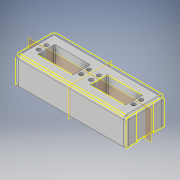
# Autodesk Inventor part: Socle servo
Saved by Autodesk Inventor 2018 (Build 220112000, 112)
## iProperties
Created: 2017-10-12
Part Number: Socle servo
Material: Generic
Document SubType Name: Modeling
Designer: liamg
Density: 1 g/cm^3
Appearance: Default
Author: liamg
Autodesk Inventor part; units mm, degrees
ref_plane "XZ Plane" through (0, 0, 0) normal (0, 1, 0) x (-1, 0, 0)
sketch "Sketch1" plane through (0, 0, 0) normal (0, 1, 0) x (-1, 0, 0)
  line L0 (-10.577, 9.85) -> (-48.827, 9.85) construction
  arc A0 (-9.577, 8.85) -> (-10.577, 9.85) centre (-10.577, 8.85) ccw construction
  line L1 (-9.577, -8.85) -> (-9.577, 8.85) construction
  arc A1 (-10.577, -9.85) -> (-9.577, -8.85) centre (-10.577, -8.85) ccw construction
  line L2 (-48.827, -9.85) -> (-10.577, -9.85) construction
  arc A2 (-49.827, -8.85) -> (-48.827, -9.85) centre (-48.827, -8.85) ccw construction
  line L3 (-49.827, 8.85) -> (-49.827, -8.85) construction
  arc A3 (-48.827, 9.85) -> (-49.827, 8.85) centre (-48.827, 8.85) ccw construction
  circle A4 centre (-19.427, 0) radius 6.44 construction
  circle A5 centre (-19.427, 0) radius 5.44 construction
  line L4 (-9.577, 9.475) -> (-3.217, 9.475) construction
  arc A6 (-2.217, 8.475) -> (-3.217, 9.475) centre (-3.217, 8.475) ccw construction
  line L5 (-2.217, -8.475) -> (-2.217, 8.475) construction
  arc A7 (-3.217, -9.475) -> (-2.217, -8.475) centre (-3.217, -8.475) ccw construction
  line L6 (-9.577, -9.475) -> (-3.217, -9.475) construction
  circle A8 centre (-5.6393, -4.36) radius 2.3 construction
  circle A9 centre (-5.6393, 4.36) radius 2.18 construction
  line L7 (-49.6076, 9.475) -> (-56.187, 9.475) construction
  arc A10 (-56.187, 9.475) -> (-57.187, 8.475) centre (-56.187, 8.475) ccw construction
  line L8 (-57.187, -8.475) -> (-57.187, 8.475) construction
  circle A11 centre (-53.7647, 4.36) radius 2.18 construction
  circle A12 centre (-53.7647, -4.36) radius 2.3 construction
  line L9 (-56.187, -9.475) -> (-49.6076, -9.475) construction
  arc A13 (-57.187, -8.475) -> (-56.187, -9.475) centre (-56.187, -8.475) ccw construction
  line L10 (48.9003, 9.85) -> (10.6503, 9.85) construction
  arc A14 (49.9003, 8.85) -> (48.9003, 9.85) centre (48.9003, 8.85) ccw construction
  line L11 (49.9003, -8.85) -> (49.9003, 8.85) construction
  arc A15 (48.9003, -9.85) -> (49.9003, -8.85) centre (48.9003, -8.85) ccw construction
  line L12 (10.6503, -9.85) -> (48.9003, -9.85) construction
  arc A16 (9.6503, -8.85) -> (10.6503, -9.85) centre (10.6503, -8.85) ccw construction
  line L13 (9.6503, 8.85) -> (9.6503, -8.85) construction
  arc A17 (10.6503, 9.85) -> (9.6503, 8.85) centre (10.6503, 8.85) ccw construction
  circle A18 centre (40.0503, 0) radius 6.44 construction
  circle A19 centre (40.0503, 0) radius 5.44 construction
  line L14 (49.9003, 9.475) -> (56.2603, 9.475) construction
  arc A20 (57.2603, 8.475) -> (56.2603, 9.475) centre (56.2603, 8.475) ccw construction
  line L15 (57.2603, -8.475) -> (57.2603, 8.475) construction
  arc A21 (56.2603, -9.475) -> (57.2603, -8.475) centre (56.2603, -8.475) ccw construction
  line L16 (49.9003, -9.475) -> (56.2603, -9.475) construction
  circle A22 centre (53.838, -4.36) radius 2.3 construction
  circle A23 centre (53.838, 4.36) radius 2.18 construction
  line L17 (9.8697, 9.475) -> (3.2903, 9.475) construction
  arc A24 (3.2903, 9.475) -> (2.2903, 8.475) centre (3.2903, 8.475) ccw construction
  line L18 (2.2903, -8.475) -> (2.2903, 8.475) construction
  circle A25 centre (5.7126, 4.36) radius 2.18 construction
  circle A26 centre (5.7126, -4.36) radius 2.3 construction
  line L19 (3.2903, -9.475) -> (9.8697, -9.475) construction
  arc A27 (2.2903, -8.475) -> (3.2903, -9.475) centre (3.2903, -8.475) ccw construction
  line L20 (-62.7873, 21.97) -> (62.7873, 21.97)
  line L21 (62.7873, 21.97) -> (62.7873, -21.97)
  line L22 (62.7873, -21.97) -> (-62.7873, -21.97)
  line L23 (-62.7873, -21.97) -> (-62.7873, 21.97)
  line L24 (-62.7873, 21.97) -> (62.7873, -21.97) construction
  line L25 (62.7873, 21.97) -> (-62.7873, -21.97) construction
  point P0 (0, 0)
  constraints: 52 end point, 32 point on circle, 28 centre point, 2 midpoint, 2 parallel, 1 horizontal, 1 perpendicular
extrude "Socle" add sketch "Sketch1" along normal blind 30
sketch "Sketch2" plane through (0, 30, 0) normal (0, 1, 0) x (1, 0, 0)
  line L0 (-10.577, 9.85) -> (-48.827, 9.85)
  arc A0 (-9.577, 8.85) -> (-10.577, 9.85) centre (-10.577, 8.85) ccw
  line L1 (-9.577, -8.85) -> (-9.577, 8.85)
  arc A1 (-10.577, -9.85) -> (-9.577, -8.85) centre (-10.577, -8.85) ccw
  line L2 (-48.827, -9.85) -> (-10.577, -9.85)
  arc A2 (-49.827, -8.85) -> (-48.827, -9.85) centre (-48.827, -8.85) ccw
  line L3 (-49.827, 8.85) -> (-49.827, -8.85)
  arc A3 (-48.827, 9.85) -> (-49.827, 8.85) centre (-48.827, 8.85) ccw
  circle A4 centre (-19.427, 0) radius 6.44 construction
  circle A5 centre (-19.427, 0) radius 5.44 construction
  line L4 (-9.577, 9.475) -> (-3.217, 9.475) construction
  arc A6 (-2.217, 8.475) -> (-3.217, 9.475) centre (-3.217, 8.475) ccw construction
  line L5 (-2.217, -8.475) -> (-2.217, 8.475) construction
  arc A7 (-3.217, -9.475) -> (-2.217, -8.475) centre (-3.217, -8.475) ccw construction
  line L6 (-9.577, -9.475) -> (-3.217, -9.475) construction
  circle A8 centre (-5.6393, -4.36) radius 2.3
  circle A9 centre (-5.6393, 4.36) radius 2.18
  line L7 (-49.6076, 9.475) -> (-56.187, 9.475) construction
  arc A10 (-56.187, 9.475) -> (-57.187, 8.475) centre (-56.187, 8.475) ccw construction
  line L8 (-57.187, -8.475) -> (-57.187, 8.475) construction
  circle A11 centre (-53.7647, 4.36) radius 2.18
  circle A12 centre (-53.7647, -4.36) radius 2.3
  line L9 (-56.187, -9.475) -> (-49.6076, -9.475) construction
  arc A13 (-57.187, -8.475) -> (-56.187, -9.475) centre (-56.187, -8.475) ccw construction
  circle A14 centre (40.0503, 0) radius 5.44 construction
  circle A15 centre (40.0503, 0) radius 6.44 construction
  line L10 (48.9003, 9.85) -> (10.6503, 9.85)
  line L11 (10.6503, -9.85) -> (48.9003, -9.85)
  arc A16 (48.9003, -9.85) -> (49.9003, -8.85) centre (48.9003, -8.85) ccw
  arc A17 (49.9003, 8.85) -> (48.9003, 9.85) centre (48.9003, 8.85) ccw
  line L12 (49.9003, -8.85) -> (49.9003, 8.85)
  circle A18 centre (53.838, 4.36) radius 2.18
  line L13 (49.9003, 9.475) -> (56.2603, 9.475) construction
  arc A19 (57.2603, 8.475) -> (56.2603, 9.475) centre (56.2603, 8.475) ccw construction
  line L14 (57.2603, -8.475) -> (57.2603, 8.475) construction
  circle A20 centre (53.838, -4.36) radius 2.3
  line L15 (49.9003, -9.475) -> (56.2603, -9.475) construction
  arc A21 (56.2603, -9.475) -> (57.2603, -8.475) centre (56.2603, -8.475) ccw construction
  arc A22 (9.6503, -8.85) -> (10.6503, -9.85) centre (10.6503, -8.85) ccw
  line L16 (9.6503, 8.85) -> (9.6503, -8.85)
  arc A23 (10.6503, 9.85) -> (9.6503, 8.85) centre (10.6503, 8.85) ccw
  line L17 (9.8697, 9.475) -> (3.2903, 9.475) construction
  circle A24 centre (5.7126, 4.36) radius 2.18
  arc A25 (3.2903, 9.475) -> (2.2903, 8.475) centre (3.2903, 8.475) ccw construction
  line L18 (2.2903, -8.475) -> (2.2903, 8.475) construction
  circle A26 centre (5.7126, -4.36) radius 2.3
  line L19 (3.2903, -9.475) -> (9.8697, -9.475) construction
  arc A27 (2.2903, -8.475) -> (3.2903, -9.475) centre (3.2903, -8.475) ccw construction
  line L20 (-62.7873, 21.97) -> (62.7873, 21.97) construction
  line L21 (62.7873, 21.97) -> (62.7873, -21.97) construction
  line L22 (62.7873, -21.97) -> (-62.7873, -21.97) construction
  line L23 (-62.7873, -21.97) -> (-62.7873, 21.97) construction
  line L24 (-62.7873, 21.97) -> (62.7873, -21.97) construction
  line L25 (62.7873, 21.97) -> (-62.7873, -21.97) construction
  point P0 (0, 0)
  point P1 (0, 0)
  point P2 (0, 0)
  constraints: 52 end point, 32 point on circle, 28 centre point, 2 midpoint, 2 parallel, 1 horizontal, 1 perpendicular
extrude "empreinte" cut sketch "Sketch2" against normal blind 28
fillet "Fillet1" radius 3.175 1 edges at (-62.7873, 15, 21.97)
fillet "Fillet2" radius 3.175 1 edges at (62.7873, 15, 21.97)
fillet "Fillet3" radius 3.175 1 edges at (62.7873, 15, -21.97)
fillet "Fillet4" radius 3.175 1 edges at (-62.7873, 15, -21.97)
chamfer "Chamfer1" distance 3.175 angle 45 8 edges at (0, 30, 21.97) (61.8574, 30, 21.0401) (62.7873, 30, 0) (61.8574, 30, -21.0401) (0, 30, -21.97) (-61.8574, 30, -21.0401) (-62.7873, 30, 0) (-61.8574, 30, 21.0401)
sketch "Sketch3" plane through (-62.7873, 0, -18.795) normal (-1, 0, 0) x (0, 0, 1)
  point P0 (18.795, 0)
sketch "Sketch4" plane through (-62.7873, 0, -18.795) normal (-1, 0, 0) x (0, 0, 1)
  line L0 (-3.175, 0) -> (-3.175, 26.825) projected
  line L1 (0, 0) -> (-3.175, 0) projected
  line L2 (0, 0) -> (37.59, 0) projected
  line L3 (40.765, 0) -> (37.59, 0) projected
  line L4 (40.765, 26.825) -> (40.765, 0) projected
  point P0 (18.795, 0)
sketch "Sketch5" plane through (-62.7873, 0, -18.795) normal (-1, 0, 0) x (0, 0, 1)
  line L0 (12.255, 30) -> (12.255, 2) construction
  line L1 (28.758, 1.5182) -> (8.832, 1.5182)
  line L2 (8.832, 1.5182) -> (8.832, 0) construction
  line L3 (8.832, 0) -> (28.758, 0) construction
  line L4 (28.758, 0) -> (28.758, 1.5182) construction
  line L5 (28.758, 1.5182) -> (8.832, 0) construction
  line L6 (8.832, 1.5182) -> (28.758, 0) construction
  line L7 (25.455, 30) -> (25.455, 2) construction
  line L8 (8.832, 1.5182) -> (10.3503, 0)
  line L9 (8.832, 1.5182) -> (10.9792, 1.5182) construction
  line L10 (28.758, 1.5182) -> (27.2397, 0)
  line L11 (28.758, 1.5182) -> (30.9051, 1.5182) construction
  line L12 (10.3503, 0) -> (27.2397, 0) construction
  line L13 (10.3503, 0) -> (27.2397, 0)
  line L14 (37.59, 0) -> (0, 0) projected
  point P0 (18.795, 0)
  point P1 (18.795, 0.7591)
  dimension "d11" = 45
  dimension "d12" = 135
  constraints: 24 end point, 4 point on line, 3 horizontal, 2 equal length, 2 midpoint, 2 parallel, 1 collinear, 1 perpendicular
  measures "d11" angle of L8 L9
  measures "d12" angle of L10 L11
extrude "Extrusion3" cut sketch "Sketch5" against normal blind 125.8875
sketch "Sketch6" plane through (62.7873, 0, -18.795) normal (1, 0, 0) x (0, 0, -1)
  line L0 (-28.758, 1.5182) -> (-8.832, 1.5182) projected
  line L1 (-8.832, 1.5182) -> (-10.3503, 0) projected
  line L2 (0, 0) -> (-10.3503, 0) projected
  line L3 (3.175, 0) -> (0, 0) projected
  line L4 (3.175, 0) -> (3.175, 26.825) projected
  line L5 (0, 30) -> (3.175, 26.825) projected
  line L6 (0, 30) -> (-37.59, 30) projected
  line L7 (-40.765, 26.825) -> (-37.59, 30) projected
  line L8 (-40.765, 26.825) -> (-40.765, 0) projected
  line L9 (-37.59, 0) -> (-40.765, 0) projected
  line L10 (-27.2397, 0) -> (-37.59, 0) projected
  line L11 (-9.945, 30) -> (-9.945, 2) projected
  line L12 (-28.645, 30) -> (-28.645, 2) projected
  line L13 (-27.2397, 0) -> (-28.758, 1.5182) projected
  point P0 (-18.795, 0)
sketch "Sketch7" plane through (59.6123, 0, -21.97) normal (0, 0, -1) x (-1, 0, 0)
  point P0 (59.6123, 0)
sketch "Sketch8" plane through (0, 30, 0) normal (0, 1, 0) x (1, 0, 0)
  line L0 (9.6503, -8.85) -> (9.6503, 8.85) projected
  line L1 (10.6503, 9.85) -> (48.9003, 9.85) projected
  line L2 (48.9003, -9.85) -> (10.6503, -9.85) projected
  line L3 (59.6123, -18.795) -> (-59.6123, -18.795) projected
  line L4 (-59.6123, -21.97) -> (59.6123, -21.97) projected
  line L5 (62.7873, 18.795) -> (62.7873, -18.795) projected
  line L6 (62.7873, -21.97) -> (62.7873, -18.795) projected
  line L7 (59.6123, 21.97) -> (-59.6123, 21.97) projected
  line L8 (-62.7873, 18.795) -> (-62.7873, -18.795) projected
  arc A0 (-59.6123, 21.97) -> (-62.7873, 18.795) centre (-59.6123, 18.795) ccw projected
  arc A1 (-62.7873, -18.795) -> (-59.6123, -21.97) centre (-59.6123, -18.795) ccw projected
  arc A2 (62.7873, 18.795) -> (59.6123, 21.97) centre (59.6123, 18.795) ccw projected
  line L9 (-10.577, -9.85) -> (-48.827, -9.85) projected
  point P0 (0, 0)
body "Solid1"
